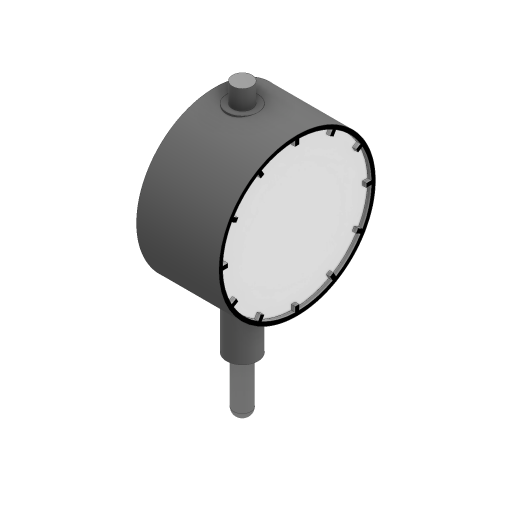
# Autodesk Inventor part: Messuhr-Dummy
Saved by Autodesk Inventor 2023.2 (Build 272271000, 271)
## iProperties
Created: 2024-12-10
Part Number: Messuhr-Dummy
Material: Generisch
Document SubType Name: Modeling
Designer: Nils Bade
Density: 1 g/cm^3
Appearance: Vorgabe
Author: Nils Bade
Autodesk Inventor part; units mm, degrees
ref_plane "YZ Plane" through (0, 0, 0) normal (1, 0, 0) x (0, 1, 0)
ref_plane "XZ Plane" through (0, 0, 0) normal (0, 1, 0) x (-1, 0, 0)
sketch "S-Pinout" plane through (0, 0, 0) normal (0, 1, 0) x (-1, 0, 0)
  circle A0 centre (0, 0) radius 4
  circle A1 centre (0, 0) radius 2.25
  dimension "d0" = 8
  dimension "d3" = 4.5
  constraints: 2 centre point, 2 coincident
  measures "d0" diameter of A0
  measures "d3" diameter of A1
extrude "Ex-passstift" add sketch "S-Pinout" along normal blind 40 and the other way blind 15 contours A0 | A1
extrude "Ex-Pin" add sketch "S-Pinout" against normal blind 14 from surface at -15 contours A1
fillet "Rundung-Pin" radius 2 1 edges at (2.25, -29, 0)
sketch "Skizze2" plane through (0, 0, 0) normal (1, 0, 0) x (0, 1, 0)
  circle A0 centre (20, 0) radius 20
  line L0 (-8, 0) -> (48, 0) construction
  line L1 (0, 28) -> (0, -28) projected
  point P0 (0, 0)
  dimension "d7" = 40
  constraints: 1 centre point, 1 midpoint, 1 tangent
  measures "d7" diameter of A0
extrude "Ex-Uhr" add sketch "Skizze2" along normal blind 14 and the other way blind 7
sketch "Skizze3" plane through (0, 40, 0) normal (0, 1, 0) x (1, 0, 0)
  circle A0 centre (0, 0) radius 0.25 projected
  circle A1 centre (0, 0) radius 2.5
  dimension "d14" = 5
  constraints: 1 centre point, 1 coincident
  measures "d14" diameter of A1
extrude "Ex-Taste" add sketch "Skizze3" along normal blind 5 contours A0 | A1
ref_plane "Messbereich" through (0, -24, 0) normal (0, -1, 0) x (1, 0, 0)
sketch "Skizze4" plane through (14, 20, 0) normal (1, 0, 0) x (0, 0, -1)
  circle A0 centre (0, 0) radius 20 projected
  circle A1 centre (0, 0) radius 20 projected
  line L0 (-0.5, 19.9937) -> (-0.5, 17.6678)
  line L1 (-0.5, 17.6678) -> (0.5, 17.6678)
  line L2 (0.5, 17.6678) -> (0.5, 19.9937)
  line L3 (0, -63.8) -> (0, 39.8) construction
  line L4 (-8.4009, 15.5508) -> (-9.5639, 17.5651)
  line L5 (-10.4299, 17.0651) -> (-9.2669, 15.0508)
  line L6 (-9.2669, 15.0508) -> (-8.4009, 15.5508)
  line L7 (-15.0508, 9.2669) -> (-17.0651, 10.4299)
  line L8 (-17.5651, 9.5639) -> (-15.5508, 8.4009)
  line L9 (-15.5508, 8.4009) -> (-15.0508, 9.2669)
  line L10 (-17.6678, 0.5) -> (-19.9937, 0.5)
  line L11 (-19.9937, -0.5) -> (-17.6678, -0.5)
  line L12 (-17.6678, -0.5) -> (-17.6678, 0.5)
  line L13 (-15.5508, -8.4009) -> (-17.5651, -9.5639)
  line L14 (-17.0651, -10.4299) -> (-15.0508, -9.2669)
  line L15 (-15.0508, -9.2669) -> (-15.5508, -8.4009)
  line L16 (-9.2669, -15.0508) -> (-10.4299, -17.0651)
  line L17 (-9.5639, -17.5651) -> (-8.4009, -15.5508)
  line L18 (-8.4009, -15.5508) -> (-9.2669, -15.0508)
  line L19 (-0.5, -17.6678) -> (-0.5, -19.9937)
  line L20 (0.5, -19.9937) -> (0.5, -17.6678)
  line L21 (0.5, -17.6678) -> (-0.5, -17.6678)
  line L22 (8.4009, -15.5508) -> (9.5639, -17.5651)
  line L23 (10.4299, -17.0651) -> (9.2669, -15.0508)
  line L24 (9.2669, -15.0508) -> (8.4009, -15.5508)
  line L25 (15.0508, -9.2669) -> (17.0651, -10.4299)
  line L26 (17.5651, -9.5639) -> (15.5508, -8.4009)
  line L27 (15.5508, -8.4009) -> (15.0508, -9.2669)
  line L28 (17.6678, -0.5) -> (19.9937, -0.5)
  line L29 (19.9937, 0.5) -> (17.6678, 0.5)
  line L30 (17.6678, 0.5) -> (17.6678, -0.5)
  line L31 (15.5508, 8.4009) -> (17.5651, 9.5639)
  line L32 (17.0651, 10.4299) -> (15.0508, 9.2669)
  line L33 (15.0508, 9.2669) -> (15.5508, 8.4009)
  line L34 (9.2669, 15.0508) -> (10.4299, 17.0651)
  line L35 (9.5639, 17.5651) -> (8.4009, 15.5508)
  line L36 (8.4009, 15.5508) -> (9.2669, 15.0508)
  circle A2 centre (0, 0) radius 19
  point P0 (0, -20)
  point P1 (-0.5, 18.9934)
  point P2 (-9.0637, 16.6988)
  point P3 (-9.9297, 16.1988)
  point P4 (-16.1988, 9.9297)
  point P5 (-16.6988, 9.0637)
  point P6 (-18.9934, 0.5)
  point P7 (-18.9934, -0.5)
  point P8 (-16.6988, -9.0637)
  point P9 (-16.1988, -9.9297)
  point P10 (-9.9297, -16.1988)
  point P11 (-9.0637, -16.6988)
  point P12 (-0.5, -18.9934)
  point P13 (0.5, -18.9934)
  point P14 (9.0637, -16.6988)
  point P15 (9.9297, -16.1988)
  point P16 (16.1988, -9.9297)
  point P17 (16.6988, -9.0637)
  point P18 (18.9934, -0.5)
  point P19 (18.9934, 0.5)
  point P20 (16.6988, 9.0637)
  point P21 (16.1988, 9.9297)
  point P22 (9.9297, 16.1988)
  point P23 (9.0637, 16.6988)
  point P24 (0.5, 18.9934)
  dimension "d18" = 1
  dimension "d21" = 360
  dimension "d23" = 1
  constraints: 72 end point, 2 point on circle, 1 horizontal, 1 perpendicular, 88 other
  measures "d18" distance of L0.end L1.end
extrude "Extrusion5" cut sketch "Skizze4" against normal blind 1 contours L29 L30 L28 A2 L26 L27 L25 L23 L24 L22 L20 L21 L19 L17 L18 L16 L14 L15 L13 L11 L12 L10 L8 L9 L7 L5 L6 L4 L0 L1 L2 L35 L36 L34 L32 L33 L31
